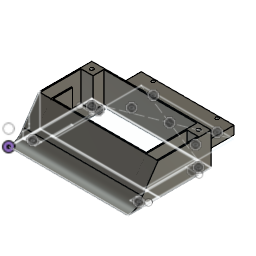
bottom (Autodesk Fusion 360 design; units mm, degrees)
part number: 2026-01-02-14-37-22-833
Autodesk Fusion 360 part; units mm, degrees
sketch "Szkic1" plane through (0, 0, 0) normal (0, 0, 1) x (1, 0, 0)
  line L0 (0, 0) -> (99, 0)
  line L1 (99, 0) -> (99, 69)
  line L2 (99, 69) -> (0, 69)
  line L3 (0, 69) -> (0, 0)
  line L4 (11, 69) -> (88, 69)
  line L5 (88, 69) -> (88, 99)
  line L6 (88, 99) -> (11, 99)
  line L7 (11, 99) -> (11, 69)
  line L8 (11, 69) -> (88, 99) construction
  line L9 (88, 69) -> (11, 99) construction
  line L10 (0, 69) -> (99, 69)
  line L11 (99, 69) -> (99, 68)
  line L12 (0, 68) -> (0, 69)
  line L13 (0, 0) -> (99, 0)
  line L14 (99, 0) -> (99, 26)
  line L15 (0, 26) -> (0, 0)
  line L16 (1, 59) -> (1, 12)
  line L17 (1, 12) -> (0, 12)
  line L18 (0, 12) -> (0, 68)
  line L19 (98, 59) -> (98, 12)
  line L20 (98, 12) -> (99, 12)
  line L21 (99, 12) -> (99, 68)
  line L22 (0, 69) -> (11, 69)
  line L23 (11, 68) -> (11, 59)
  line L24 (11, 59) -> (1, 59)
  line L25 (0, 59) -> (0, 69)
  line L26 (88, 68) -> (88, 59)
  line L27 (89, 59) -> (98, 59)
  line L28 (99, 59) -> (99, 69)
  line L29 (88, 68) -> (11, 68)
  line L30 (89, 59) -> (89, 26)
  line L31 (89, 26) -> (88, 26)
  line L32 (88, 26) -> (88, 59)
  line L33 (11, 59) -> (10, 59)
  line L34 (11, 26) -> (10, 26)
  line L35 (10, 26) -> (10, 42)
  line L36 (10, 42) -> (11, 42)
  line L37 (11, 42) -> (11, 26)
  line L38 (11, 26) -> (89, 26)
  line L39 (89, 26) -> (89, 25)
  line L40 (89, 25) -> (10, 25)
  line L41 (10, 25) -> (10, 26)
  line L42 (11, 68) -> (13, 68)
  line L43 (13, 68) -> (13, 26)
  line L44 (13, 26) -> (11, 26)
  line L45 (11, 26) -> (11, 68)
  line L46 (88, 68) -> (86, 68)
  line L47 (86, 68) -> (86, 26)
  line L48 (86, 26) -> (88, 26)
  line L49 (88, 26) -> (88, 68)
  line L50 (1, 12) -> (10, 12)
  line L51 (10, 12) -> (10, 26)
  line L52 (10, 26) -> (1, 26)
  line L53 (1, 26) -> (1, 12)
  line L54 (1, 12) -> (10, 12)
  line L55 (10, 12) -> (10, 17)
  line L56 (10, 17) -> (1, 17)
  line L57 (1, 17) -> (1, 12)
  circle A0 centre (5.5, 14.5) radius 0.9
  line L58 (99, 26) -> (11, 26)
  line L59 (10, 26) -> (0, 26)
  line L60 (89, 26) -> (98, 26)
  line L61 (98, 26) -> (98, 18)
  line L62 (89, 26) -> (98, 26)
  line L63 (98, 26) -> (98, 17)
  line L64 (98, 17) -> (89, 17)
  line L65 (89, 17) -> (89, 26)
  line L66 (89, 17) -> (98, 17)
  line L67 (98, 17) -> (98, 12)
  line L68 (98, 12) -> (89, 12)
  line L69 (89, 12) -> (89, 17)
  circle A1 centre (93.5, 14.5) radius 0.9
  circle A2 centre (23, 97) radius 1.4
  circle A3 centre (23, 79) radius 1.4
  circle A4 centre (76, 79) radius 1.4
  circle A5 centre (76, 97) radius 1.4
  circle A6 centre (5.5, 63.5) radius 1.5
  circle A7 centre (93.5, 64) radius 1.5
  point P0 (49.5, 84)
  point P1 (49.5, 84)
  point P2 (5.5, 14.5)
  point P3 (93.5, 14.5)
  point P4 (76, 79)
  point P5 (76, 97)
  point P6 (23, 97)
  point P7 (23, 79)
  point P8 (11, 63.5)
  point P9 (5.5, 63.5)
  point P10 (93.5, 59)
  point P11 (93.5, 64)
  dimension "d1" = 99
  dimension "d2" = 69
  dimension "d4" = 77
  dimension "d5" = 1
  dimension "d6" = 26
  dimension "d8" = 56
  dimension "d10" = 56
  dimension "d11" = 11
  dimension "d12" = 10
  dimension "d13" = 10
  dimension "d14" = 1
  dimension "d15" = 16
  dimension "d17" = 1.8
  dimension "d19" = 9
  dimension "d20" = 1.8
  dimension "d25" = 2.8
  dimension "d26" = 2.8
  dimension "d27" = 2.8
  dimension "d28" = 2.8
  dimension "d56" = 3
  dimension "d57" = 3
  dimension "d61" = 30
  dimension "d62" = 2
  dimension "d64" = 10
  dimension "d65" = 12
  dimension "d66" = 10
  dimension "d67" = 2
  dimension "d68" = 12
  dimension "d69" = 12
  dimension "d70" = 2
  dimension "d71" = 12
  dimension "d72" = 10
  dimension "d73" = 5
  dimension "d74" = 5.5
  dimension "d75" = 5.5
  dimension "d76" = 5.5
  dimension "d77" = 4.5
  dimension "d78" = 2.5
  dimension "d79" = 4.5
  dimension "d80" = 2.5
  constraint horizontal L0
  constraint vertical L1
  constraint horizontal L2
  constraint vertical L3
  constraint coincident L0.start L3.end
  constraint horizontal L4
  constraint perpendicular L4 L5
  constraint parallel L4 L6
  constraint parallel L5 L7
  constraint coincident L8 P1
  constraint coincident L9 P1
  constraint coincident P1 P0
  constraint horizontal L10
  constraint vertical L11
  constraint vertical L12
  constraint horizontal L13
  constraint vertical L14
  constraint horizontal L58
  constraint vertical L15
  constraint coincident L1 L14.end
  constraint vertical L16
  constraint horizontal L17
  constraint vertical L18
  constraint vertical L19
  constraint horizontal L20
  constraint vertical L21
  constraint horizontal L22
  constraint vertical L23
  constraint horizontal L24
  constraint vertical L25
  constraint vertical L26
  constraint horizontal L27
  constraint vertical L28
  constraint vertical L30
  constraint horizontal L31
  constraint vertical L32
  constraint horizontal L33
  constraint coincident L34.end L58
  constraint horizontal L34
  constraint vertical L35
  constraint horizontal L36
  constraint vertical L37
  constraint horizontal L38
  constraint vertical L39
  constraint horizontal L40
  constraint vertical L41
  constraint horizontal L42
  constraint vertical L43
  constraint horizontal L44
  constraint vertical L45
  constraint coincident L38 L43.end
  constraint horizontal L46
  constraint vertical L47
  constraint horizontal L48
  constraint vertical L49
  constraint coincident L47.end L58
  constraint horizontal L50
  constraint vertical L51
  constraint horizontal L52
  constraint vertical L53
  constraint horizontal L54
  constraint vertical L55
  constraint horizontal L56
  constraint vertical L57
  constraint coincident L51 L55.end
  constraint coincident P2 A0.centre
  constraint collinear L58 L59
  constraint horizontal L60
  constraint vertical L61
  constraint horizontal L62
  constraint vertical L63
  constraint horizontal L64
  constraint vertical L65
  constraint horizontal L66
  constraint vertical L67
  constraint horizontal L68
  constraint vertical L69
  constraint coincident P3 A1.centre
  constraint coincident P6 A2.centre
  constraint coincident P7 A3.centre
  constraint coincident P4 A4.centre
  constraint coincident P5 A5.centre
  constraint midpoint L23 P8
  constraint coincident P9 A6.centre
  constraint midpoint L27 P10
  constraint coincident P11 A7.centre
  constraint equal L24 L25
  constraint collinear L17 L20
  constraint equal L11 L17
  constraint coincident L2 L4.start
  constraint coincident L1 L11.end
  constraint equal L24 L59
  constraint coincident L4.start L7.end
  constraint collinear L24 L27
  constraint equal L11 L20
  constraint equal L11 L31
  constraint equal L11 L33
  constraint equal L11 L34
  constraint equal L11 L39
  constraint equal L4 L29
  constraint coincident L34.end L35.start
  constraint equal L23 L26
  constraint equal L23 L27
  constraint equal L23 L60
  constraint equal L23 L64
  constraint equal L23 L66
  constraint equal L55 L67
  constraint collinear L31 L34
  constraint equal L43 L47
  constraint equal L42 L46
  measures "d1" distance of L0.start L0.end
  measures "d2" distance of L0.start L2.end
  measures "d4" distance of L5.end L6.end
  measures "d5" distance of L2.end L12.start
  measures "d6" distance of L0.start L15.start
  measures "d8" distance of L12.start L17.end
  measures "d10" distance of L11.end L20.end
  measures "d11" distance of L2.end L4.start
  measures "d12" distance of L2.end L25.start
  measures "d13" distance of L1.end L28.start
  measures "d14" distance of L26.end L27.start
  measures "d15" distance of L34.start L36.end
  measures "d17" diameter of A0
  measures "d19" distance of L30.end L64.end
  measures "d20" diameter of A1
  measures "d25" diameter of A2
  measures "d26" diameter of A3
  measures "d27" diameter of A4
  measures "d28" diameter of A5
  measures "d56" diameter of A6
  measures "d57" diameter of A7
  measures "d61" distance of L4.end L5.end
  measures "d62" distance of L43 L45
  measures "d64" distance of L2 L24
  measures "d65" distance of L7 P7
  measures "d66" distance of L10 P7
  measures "d67" distance of L6 P6
  measures "d68" distance of L7 P6
  measures "d69" distance of L5 P5
  measures "d70" distance of L6 P5
  measures "d71" distance of L5 P4
  measures "d72" distance of L10 P4
  measures "d73" distance of L10 P11
  measures "d74" distance of L1 P11
  measures "d75" distance of L10 P9
  measures "d76" distance of L25 P9
  measures "d77" distance of L57 P2
  measures "d78" distance of L56 P2
  measures "d79" distance of L67 P3
  measures "d80" distance of L64 P3
extrude "Wyciągnięcie proste1" add sketch "Szkic1" along normal blind 27 contours L1 L2 L3 L4 L10 L11 L12 L16 L18 L19 L21 L22 L23 L24 L25 L26 L27 L28 L29 L30 L31 L32 L33 L38 L42 L45 L46 L49 L58 L59 | L34 L35 L36 L37 L45 | L31 L34 L38 L39 L40 L41 L44 L48 L51 L58 L65 | A6 | A7 makes body 1
extrude "Wyciągnięcie proste2" add sketch "Szkic1" along normal blind 2 separate body contours L16 L24 L33 L35 L36 L45 L52 L59 | L19 L27 L30 L58 L60 L62 | L23 L29 L37 L38 L42 L43 L44 L45 L58 | L26 L29 L32 L38 L46 L47 L48 L49 L58 makes body 2 at (4, 42.3333, 0) makes body 3 at (86.6667, 40, 0) makes body 4 at (95, 37, 0)
extrude "Wyciągnięcie proste3" add sketch "Szkic1" along normal blind 7 from surface at 3 contours L2 L4 L5 L6 L7 L10 bodies 1
extrude "Wyciągnięcie proste4" add sketch "Szkic1" along normal blind 3 separate body contours L16 L50 L51 L53 L54 L55 L56 L57 | L19 L64 L66 L67 L68 L69 makes body 5 at (90.2, 14.5, 0) makes body 6 at (2.2, 14.5, 0)
combine "Kombinacja1" operation add target body 1 tool bodies 2 3 4
sketch "Szkic2" plane through (0, 0, 0) normal (1, 0, 0) x (0, 1, 0)
  line L0 (0, 0) -> (12, 0)
  line L1 (12, 0) -> (12, 5)
  arc A0 (0, 0) -> (12, 8) centre (0, 13) ccw
  line L2 (17, 8) -> (17, 5)
  line L3 (17, 5) -> (12, 5)
  line L4 (12, 8) -> (25, 27)
  line L5 (17, 8) -> (17, 14.3077)
  line L6 (25, 27) -> (25, 26)
  line L7 (25, 26) -> (17, 14.3077)
  line L8 (25, 27) -> (26, 27)
  line L9 (26, 27) -> (26, 0)
  line L10 (26, 0) -> (0, 0)
  dimension "d38" = 12
  dimension "d40" = 5
  dimension "d41" = 3
  dimension "d42" = 1
  dimension "d81" = 13
  dimension "d82" = 27
  dimension "d83" = 26
  constraint horizontal L0
  constraint vertical L1
  constraint coincident L0.start A0.start
  constraint tangent L0 A0
  constraint vertical L2
  constraint horizontal L3
  constraint vertical L6
  constraint parallel L4 L7
  constraint perpendicular L6 L8
  constraint perpendicular L8 L9
  constraint tangent A0 L10
  constraint perpendicular L9 L10
  constraint parallel L5 L9
  constraint equal L6 L8
  constraint equal L1 L3
  measures "d38" distance of L0.start L0.end
  measures "d40" distance of A0.end L2.start
  measures "d41" distance of A0.end L1.end
  measures "d42" distance of L4.end L6.end
  measures "d81" radius of A0
  measures "d82" distance of L8 L10
  measures "d83" distance of A0.centre L9
extrude "Wyciągnięcie proste5" add sketch "Szkic2" along normal blind 10 contours L0 L1 A0 L2 L3 L4 L5 L6 L7 L10 bodies 1 6
extrude "Wyciągnięcie proste6" add sketch "Szkic2" along normal blind 9 from surface at 89 contours L0 L1 A0 L2 L3 L4 L5 L6 L7 L10 bodies 1 5
extrude "Wyciągnięcie proste7" add sketch "Szkic2" along normal blind 1 bodies 1
extrude "Wyciągnięcie proste8" add sketch "Szkic2" along normal blind 1 from surface at 98 bodies 1
extrude "Wyciągnięcie proste9" add sketch "Szkic2" along normal blind 79 from surface at 10 bodies 1
extrude "Wyciągnięcie proste10" cut sketch "Szkic1" along normal blind 11 from surface at 16 contours A6 | A7 bodies 1
